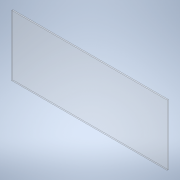
# Autodesk Inventor part: Acrilico1_Prensa
Saved by Autodesk Inventor 2021 (Build 250183000, 183)
## iProperties
Created: 2021-08-02
Part Number: Acrilico1_Prensa
Material: PMMA Plastic
Document SubType Name: Modeling
Designer: Nelson
Density: 1.188 g/cm^3
Appearance: Polycarbonate - Clear
Author: Nelson
Autodesk Inventor part; units mm, degrees
ref_plane "YZ Plane" through (0, 0, 0) normal (1, 0, 0) x (0, 1, 0)
ref_plane "XZ Plane" through (0, 0, 0) normal (0, 1, 0) x (-1, 0, 0)
ref_plane "XY Plane" through (0, 0, 0) normal (0, 0, 1) x (1, 0, 0)
sketch "Sketch1" plane through (0, 0, 0) normal (0, 0, 1) x (1, 0, 0)
  line L0 (1250.8, 0) -> (1250.8, 489.6)
  line L1 (1250.8, 489.6) -> (0, 489.6)
  line L2 (0, 489.6) -> (0, 0)
  line L3 (0, 0) -> (362, 0)
  line L4 (0, 0) -> (1250.8, 0)
  dimension "d0" = 1250.8
  dimension "d1" = 489.6
  constraints: 10 end point, 2 horizontal, 2 parallel
  measures "d0" distance of L1.end L0.end
  measures "d1" distance of L0.start L0.end
extrude "Extrusion1" add sketch "Sketch1" against normal blind 10
body "Solid1"
